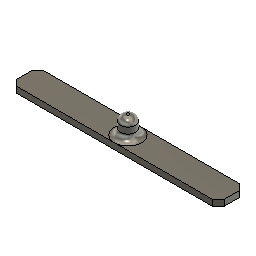
spring (Autodesk Fusion 360 design; units mm, degrees)
Autodesk Fusion 360 part; units mm, degrees
sketch "Sketch2" plane through (0, 0, 0) normal (0, 1, 0) x (1, 0, 0)
  line L0 (-34.5, -4.5) -> (34.5, -4.5)
  line L1 (34.5, -4.5) -> (34.5, 4.5)
  line L2 (34.5, 4.5) -> (-34.5, 4.5)
  line L3 (-34.5, 4.5) -> (-34.5, -4.5)
  line L4 (-34.5, -4.5) -> (34.5, 4.5) construction
  line L5 (34.5, -4.5) -> (-34.5, 4.5) construction
  circle A0 centre (0, 0) radius 2.5
  dimension "d1" = 69
  dimension "d2" = 9
  dimension "d3" = 5
  measures "d3" diameter of A0
extrude "Extrude1" add sketch "Sketch2" along normal blind 2 contours L0 L1 L2 L3 | A0 makes body 1
sketch "Sketch3" plane through (0, 2, 0) normal (0, 1, 0) x (-1, 0, 0)
  line L0 (34.5, -4.5) -> (34.5, 4.5)
  line L1 (34.5, 4.5) -> (-34.5, 4.5)
  line L2 (-34.5, 4.5) -> (-34.5, -4.5)
  line L3 (-34.5, -4.5) -> (34.5, -4.5)
  circle A0 centre (0, 0) radius 2.5
  circle A1 centre (0, 0) radius 2.5
extrude "Extrude3" add sketch "Sketch3" along normal blind 6 contours A0 A1 bodies 1
fillet "Fillet3" radius 2 1 edges at (2.3308, 2, 0.904) on bodies 1
fillet "Fillet4" radius 2 1 edges at (2.3308, 8, -0.904) on bodies 1
chamfer "Chamfer2" distance 2 angle 45 4 edges at (34.5, 1, 4.5) (34.5, 1, -4.5) (-34.5, 1, -4.5) (-34.5, 1, 4.5) on bodies 1
copy_body "Body->Comp1" bodies 1 removing the originals makes body 2 in component "spring"
component "spring" placed x (1, 0, 0) y (0, 1, 0) z (0, 0, 1) at (0, 0, 0)
equation "d4 = spring_thickness"
equation "d15 = post_length"
equation "spring_thickness = 2 mm"
equation "post_length = 6 mm"
